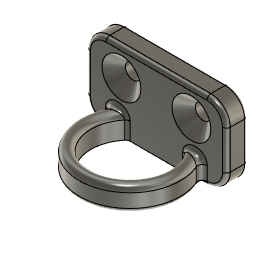
air hose hook (Autodesk Fusion 360 design; units mm, degrees)
Autodesk Fusion 360 part; units mm, degrees
sketch "Sketch1" plane through (0, 0, 0) normal (0, 0, 1) x (1, 0, 0)
  circle A0 centre (0, 0) radius 12.7
  circle A1 centre (0, 0) radius 16.51
  line L0 (-22.86, 8.6578) -> (22.86, 8.6578)
  line L1 (22.86, 8.6578) -> (22.86, 15.24)
  line L2 (22.86, 15.24) -> (-22.86, 15.24)
  line L3 (-22.86, 15.24) -> (-22.86, 8.6578)
  dimension "d1" = 25.4
  dimension "d2" = 33.02
  constraint coincident A0.centre A1.centre
  constraint concentric A0 A1
  constraint horizontal L0
  constraint vertical L1
  constraint horizontal L2
  constraint vertical L3
  measures "d1" diameter of A0
  measures "d2" diameter of A1
extrude "Extrude1" add sketch "Sketch1" along normal blind 25.4 contours A0 L0 | A0 A1 L0 L2 | A1 L0 L1 L2 | A1 L0 L2 L3 picked at (2.6337, 9.0862)
extrude "Extrude2" add sketch "Sketch1" along normal blind 7.62 contours A0 A1 L0
fillet "Fillet1" radius 1.905 2 edges at (0, -16.51, 7.62) (0, -12.7, 7.62)
fillet "Fillet2" radius 6.35 4 edges at (-22.86, 11.9489, 25.4) (22.86, 11.9489, 25.4) (-22.86, 11.9489, 0) (22.86, 11.9489, 0)
sketch "Sketch2" plane through (0, 8.6578, 0) normal (0, -1, 0) x (1, 0, 0)
  arc A0 (16.51, 0) -> (22.86, 6.35) centre (16.51, 6.35) ccw
  line L0 (22.86, 6.35) -> (22.86, 19.05)
  arc A1 (22.86, 19.05) -> (16.51, 25.4) centre (16.51, 19.05) ccw
  line L1 (16.51, 25.4) -> (-16.51, 25.4)
  arc A2 (-16.51, 25.4) -> (-22.86, 19.05) centre (-16.51, 19.05) ccw
  line L2 (-22.86, 19.05) -> (-22.86, 6.35)
  arc A3 (-22.86, 6.35) -> (-16.51, 0) centre (-16.51, 6.35) ccw
  line L3 (-16.51, 0) -> (-14.0578, 0)
  line L4 (-14.0578, 0) -> (-14.0578, 5.715)
  spline S0 degree 3 poles (-14.0578, 5.715) (-14.0578, 5.9369) (-14, 6.1969) (-13.8088, 6.6188) (-13.6345, 6.8501) (-13.2548, 7.1936) (-12.9743, 7.3574) (-12.4328, 7.5591) (-12.0693, 7.62) (-11.7621, 7.62) knots 0 0 0 0 0.066574 0.066574 0.138969 0.138969 0.220186 0.220186 0.312327 0.312327 0.312327 0.312327
  spline S1 degree 3 poles (-11.7621, 7.62) (-11.4444, 7.62) (-11.0685, 7.5557) (-10.4904, 7.3512) (-10.1793, 7.1813) (-9.7584, 6.8297) (-9.5628, 6.5975) (-9.3546, 6.1789) (-9.2915, 5.9294) (-9.2915, 5.715) knots 0.312327 0.312327 0.312327 0.312327 0.407659 0.407659 0.49628 0.49628 0.572191 0.572191 0.636524 0.636524 0.636524 0.636524
  line L5 (-9.2915, 5.715) -> (-9.2915, 0)
  line L6 (-9.2915, 0) -> (9.2915, 0)
  line L7 (9.2915, 0) -> (9.2915, 5.715)
  spline S2 degree 3 poles (9.2915, 5.715) (9.2915, 5.9294) (9.3546, 6.1789) (9.5628, 6.5975) (9.7584, 6.8297) (10.1793, 7.1813) (10.4904, 7.3512) (11.0685, 7.5557) (11.4444, 7.62) (11.7621, 7.62) knots 0.636524 0.636524 0.636524 0.636524 0.700856 0.700856 0.776767 0.776767 0.865388 0.865388 0.96072 0.96072 0.96072 0.96072
  spline S3 degree 3 poles (11.7621, 7.62) (12.0693, 7.62) (12.4328, 7.5591) (12.9743, 7.3574) (13.2548, 7.1936) (13.6345, 6.8501) (13.8088, 6.6188) (14, 6.1969) (14.0578, 5.9369) (14.0578, 5.715) knots 0.96072 0.96072 0.96072 0.96072 1.052861 1.052861 1.134078 1.134078 1.206473 1.206473 1.273047 1.273047 1.273047 1.273047
  line L8 (14.0578, 5.715) -> (14.0578, 0)
  line L9 (14.0578, 0) -> (16.51, 0)
  circle A4 centre (-11.43, 16.51) radius 2.54
  circle A5 centre (11.43, 16.51) radius 2.54
  dimension "d11" = 5.08
  dimension "d21" = 5.08
  measures "d11" diameter of A4
  measures "d21" diameter of A5
extrude "Extrude3" cut sketch "Sketch2" against normal blind 17.78 contours A4 | A5
chamfer "Chamfer1" distance 3.81 angle 45 1 edges at (-13.7981, 8.6578, 17.4285)
chamfer "Chamfer1" distance 3.81 angle 45 1 edges at (9.0619, 8.6578, 17.4285)
fillet "Fillet3" radius 1.27 10 edges at (-15.2839, 8.6578, 0) (-21.0001, 8.6578, 1.8599) (-22.86, 8.6578, 12.7) (-21.0001, 8.6578, 23.5401) (0, 8.6578, 25.4) (21.0001, 8.6578, 23.5401) (22.86, 8.6578, 12.7) (21.0001, 8.6578, 1.8599) (15.2839, 8.6578, 0) (0, -16.51, 0)
fillet "Fillet4" radius 0.635 8 edges at (21.0001, 15.24, 23.5401) (0, 15.24, 25.4) (-21.0001, 15.24, 23.5401) (-22.86, 15.24, 12.7) (-21.0001, 15.24, 1.8599) (0, 15.24, 0) (21.0001, 15.24, 1.8599) (22.86, 15.24, 12.7)
fillet "Fillet5" radius 1.5494 10 edges at (-13.2139, 9.1151, 0.2941) (-14.0578, 8.6578, 3.4925) (-13.3183, 8.6578, 7.1244) (-10.1339, 8.6578, 7.1277) (-9.2915, 8.6578, 2.8575) (9.2915, 8.6578, 2.8575) (10.1339, 8.6578, 7.1277) (13.3183, 8.6578, 7.1244) (14.0578, 8.6578, 3.4925) (13.2139, 9.1151, 0.2941)
